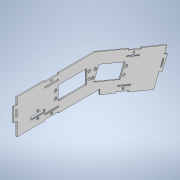
# Autodesk Inventor part: centralFinal
Saved by Autodesk Inventor 2020 (Build 240168000, 168)
## iProperties
Created: 2019-06-16
Part Number: centralFinal
Material: Generic
Document SubType Name: Modeling
Designer: Vivek Muskan
Density: 1 g/cm^3
Appearance: Default
Author: Vivek Muskan
Autodesk Inventor part; units mm, degrees
ref_plane "YZ Plane" through (0, 0, 0) normal (1, 0, 0) x (0, 1, 0)
ref_plane "XZ Plane" through (0, 0, 0) normal (0, 1, 0) x (-1, 0, 0)
ref_plane "XY Plane" through (0, 0, 0) normal (0, 0, 1) x (1, 0, 0)
sketch "Sketch1" plane through (0, 0, 0) normal (1, 0, 0) x (0, 1, 0)
  line L0 (12, -9) -> (2, -9)
  line L1 (2, -9) -> (2, 41)
  line L2 (2, 41) -> (7, 41)
  line L3 (7, 41) -> (7, 31)
  line L4 (7, 31) -> (12, 31)
  line L5 (12, 31) -> (12, -9)
  line L6 (2, 111) -> (12, 111)
  line L7 (12, 111) -> (12, 71)
  line L8 (12, 71) -> (7, 71)
  line L9 (7, 71) -> (7, 61)
  line L10 (7, 61) -> (2, 61)
  line L11 (2, 61) -> (2, 111)
  line L12 (7, 54.5) -> (7, 55)
  line L13 (7, 55) -> (62, 55)
  arc A0 (64, 57) -> (62, 55) centre (64, 55) ccw
  line L14 (64, 57) -> (65, 57)
  arc A1 (67, 55) -> (65, 57) centre (65, 55) ccw
  line L15 (67, 55) -> (102, 55)
  arc A2 (104, 57) -> (102, 55) centre (104, 55) ccw
  line L16 (104, 57) -> (105, 57)
  arc A3 (107, 55) -> (105, 57) centre (105, 55) ccw
  line L17 (107, 55) -> (107, 47)
  arc A4 (105, 45) -> (107, 47) centre (105, 47) ccw
  line L18 (105, 45) -> (104, 45)
  arc A5 (102, 47) -> (104, 45) centre (104, 47) ccw
  line L19 (102, 47) -> (67, 47)
  arc A6 (65, 45) -> (67, 47) centre (65, 47) ccw
  line L20 (65, 45) -> (64, 45)
  arc A7 (62, 47) -> (64, 45) centre (64, 47) ccw
  line L21 (62, 47) -> (7, 47)
  line L22 (7, 47) -> (7, 47.5)
  line L23 (7, 47.5) -> (-5, 47.5)
  line L24 (-5, 47.5) -> (-5, 41)
  line L25 (-5, 41) -> (0, 41)
  line L26 (0, 41) -> (0, 2.0396)
  line L27 (0, 2.0396) -> (0.3922, 1.9612)
  line L28 (0.3922, 1.9612) -> (0, 1.0198)
  line L29 (0, 1.0198) -> (0, 0)
  line L30 (0, 0) -> (-0.3922, 0.0784)
  line L31 (-0.3922, 0.0784) -> (-15.377, -35.885)
  line L32 (-15.377, -35.885) -> (-19.9924, -33.9619)
  line L33 (-19.9924, -33.9619) -> (-22.4924, -39.9619)
  line L34 (-22.4924, -39.9619) -> (-11.4155, -44.5773)
  line L35 (-11.4155, -44.5773) -> (-11.2232, -44.1158)
  line L36 (-11.2232, -44.1158) -> (39.5461, -65.2696)
  arc A8 (42.1615, -64.1927) -> (39.5461, -65.2696) centre (41.3922, -66.0388) ccw
  line L37 (42.1615, -64.1927) -> (43.0845, -64.5773)
  arc A9 (44.1615, -67.1927) -> (43.0845, -64.5773) centre (42.3153, -66.4235) ccw
  line L38 (44.1615, -67.1927) -> (76.4692, -80.6542)
  arc A10 (79.0845, -79.5773) -> (76.4692, -80.6542) centre (78.3153, -81.4235) ccw
  line L39 (79.0845, -79.5773) -> (80.0076, -79.9619)
  arc A11 (81.0845, -82.5773) -> (80.0076, -79.9619) centre (79.2384, -81.8081) ccw
  line L40 (81.0845, -82.5773) -> (78.0076, -89.9619)
  arc A12 (75.3922, -91.0388) -> (78.0076, -89.9619) centre (76.1615, -89.1927) ccw
  line L41 (75.3922, -91.0388) -> (74.4692, -90.6542)
  arc A13 (73.3922, -88.0388) -> (74.4692, -90.6542) centre (75.2384, -88.8081) ccw
  line L42 (73.3922, -88.0388) -> (41.0845, -74.5773)
  arc A14 (38.4692, -75.6542) -> (41.0845, -74.5773) centre (39.2384, -73.8081) ccw
  line L43 (38.4692, -75.6542) -> (37.5461, -75.2696)
  arc A15 (36.4692, -72.6542) -> (37.5461, -75.2696) centre (38.3153, -73.4235) ccw
  line L44 (36.4692, -72.6542) -> (-14.3001, -51.5004)
  line L45 (-14.3001, -51.5004) -> (-14.1078, -51.0388)
  line L46 (-14.1078, -51.0388) -> (-25.1847, -46.4235)
  line L47 (-25.1847, -46.4235) -> (-27.6847, -52.4235)
  line L48 (-27.6847, -52.4235) -> (-23.0693, -54.3465)
  line L49 (-23.0693, -54.3465) -> (-38.8385, -92.1927)
  line L50 (-38.8385, -92.1927) -> (-47.3001, -86.5004)
  line L51 (-47.3001, -86.5004) -> (-30.377, -45.885)
  line L52 (-30.377, -45.885) -> (-39.6078, -42.0388)
  line L53 (-39.6078, -42.0388) -> (-35.7616, -32.8081)
  line L54 (-35.7616, -32.8081) -> (-26.5308, -36.6542)
  line L55 (-26.5308, -36.6542) -> (-10, 3.0198)
  line L56 (-10, 3.0198) -> (-10, 46)
  line L57 (-10, 46) -> (-20, 46)
  line L58 (-20, 46) -> (-20, 56)
  line L59 (-20, 56) -> (-10, 56)
  line L60 (-10, 56) -> (-10, 100)
  line L61 (-10, 100) -> (0, 102)
  line L62 (0, 102) -> (0, 61)
  line L63 (0, 61) -> (-5, 61)
  line L64 (-5, 61) -> (-5, 54.5)
  line L65 (-5, 54.5) -> (7, 54.5)
  line L66 (0, 51) -> (107, 51)
  line L67 (79.5461, -86.2696) -> (-37.6847, -37.4235)
  constraints: 136 end point, 32 point on circle, 16 centre point, 3 midpoint
sketch "Sketch2" plane through (0, 0, 0) normal (1, 0, 0) x (0, 1, 0)
  line L0 (0, 0) -> (0, 51)
  line L1 (0, 51) -> (15, 51)
  line L2 (15, 51) -> (15, 101)
  line L3 (15, 101) -> (65, 101)
  line L4 (101.707, 46.9392) -> (84.707, 46.9392)
  line L5 (84.707, 46.9392) -> (34.707, 46.9392)
  line L6 (15, 51) -> (15, 60)
  line L7 (0, 0) -> (0, 1)
  line L8 (0, 1) -> (110.5886, -21.1178)
  line L9 (50.3822, 41.5) -> (30.3822, 41.5)
  line L10 (30.3822, 41.5) -> (30.3822, 0.5)
  line L11 (30.3822, 0.5) -> (50.3822, 0.5)
  line L12 (50.3822, 0.5) -> (50.3822, 41.5)
  line L13 (50.3822, 0.5) -> (45.3822, 0.5)
  line L14 (45.3822, 0.5) -> (45.3822, -3.5)
  line L15 (45.3822, -3.5) -> (35.3822, -3.5)
  circle A0 centre (45.3822, -3.5) radius 2
  circle A1 centre (35.3822, -3.5) radius 2
  line L16 (50.3822, 21) -> (30.3822, 21)
  circle A2 centre (45.3822, 45.5) radius 2
  circle A3 centre (35.3822, 45.5) radius 2
  line L17 (65, 101) -> (65, -12.0001)
  line L18 (0, 51) -> (107.1279, 51)
  line L19 (65, 51) -> (55, 51)
  line L20 (15, 51) -> (25, 51)
  line L21 (-5.3847, -50.9231) -> (-24.6156, -97.0769)
  line L22 (-24.6156, -97.0769) -> (21.5382, -116.3077)
  line L23 (21.5382, -116.3077) -> (65, -12.0001)
  line L24 (15, 51) -> (15, -19)
  line L25 (-5.3847, -50.9231) -> (7.9166, -19)
  line L26 (15, -19) -> (7.9166, -19)
  line L27 (30.9296, -55.7624) -> (12.468, -48.0701)
  line L28 (12.468, -48.0701) -> (28.2374, -10.224)
  line L29 (28.2374, -10.224) -> (46.6989, -17.9163)
  line L30 (46.6989, -17.9163) -> (30.9296, -55.7624)
  circle A4 centre (43.622, -12.3009) radius 2
  circle A5 centre (34.3912, -8.4548) radius 2
  circle A6 centre (24.7757, -57.5317) radius 2
  circle A7 centre (15.545, -53.6855) radius 2
  line L31 (65, 51) -> (65, 41)
  line L32 (65, 41) -> (63.5, 41)
  line L33 (63.5, 41) -> (63.5, 61)
  line L34 (63.5, 61) -> (65, 61)
  line L35 (65, 61) -> (65, 41)
  line L36 (63.5, 61) -> (57.5, 61)
  line L37 (57.5, 61) -> (56, 61)
  line L38 (56, 61) -> (56, 41)
  line L39 (56, 41) -> (57.5, 41)
  line L40 (57.5, 41) -> (57.5, 61)
  line L41 (65, 51) -> (60.5, 51)
  circle A8 centre (60.5, 51) radius 1.5
  line L42 (44.6152, -60.9232) -> (43.2306, -60.3463)
  line L43 (43.2306, -60.3463) -> (35.5383, -78.8078)
  line L44 (35.5383, -78.8078) -> (36.9229, -79.3847)
  line L45 (29.9998, -76.5001) -> (28.6152, -75.9231)
  line L46 (28.6152, -75.9231) -> (36.3076, -57.4616)
  line L47 (36.3076, -57.4616) -> (37.6922, -58.0386)
  line L48 (37.6922, -58.0386) -> (29.9998, -76.5001)
  circle A9 centre (36.6152, -68.4232) radius 1.5
  line L49 (-1.5387, -106.6923) -> (40, -7)
  line L50 (40, 101) -> (40, -7)
  line L51 (40, -68.0997) -> (40, -71.9997)
  circle A10 centre (-1.2309, -52.6538) radius 1.5
  line L52 (5.3845, -44.5769) -> (-2.3078, -63.0385)
  line L53 (-0.9232, -63.6154) -> (6.7691, -45.1539)
  line L54 (6.7691, -45.1539) -> (5.3845, -44.5769)
  line L55 (-2.3078, -63.0385) -> (-0.9232, -63.6154)
  line L56 (-0.1539, -42.2692) -> (-7.8463, -60.7308)
  line L57 (-7.8463, -60.7308) -> (-9.2309, -60.1538)
  line L58 (-1.5386, -41.6923) -> (-0.1539, -42.2692)
  line L59 (15, 41) -> (16.5, 41)
  line L60 (16.5, 41) -> (16.5, 61)
  line L61 (16.5, 61) -> (15, 61)
  line L62 (22.5, 61) -> (24, 61)
  line L63 (24, 61) -> (24, 41)
  line L64 (24, 41) -> (22.5, 41)
  line L65 (22.5, 41) -> (22.5, 61)
  circle A11 centre (19.5, 51) radius 1.5
  dimension "d0" = 51
  dimension "d1" = 15
  dimension "d2" = 50
  dimension "d3" = 50
  dimension "d11" = 17
  dimension "d12" = 50
  dimension "d23" = 9
  dimension "d34" = 1
  dimension "d35" = 78.69
  dimension "d36" = 20
  dimension "d37" = 41
  dimension "d38" = 5
  dimension "d39" = 4
  dimension "d40" = 10
  dimension "d41" = 4
  dimension "d42" = 4
  dimension "d43" = 10
  dimension "d47" = 10
  dimension "d48" = 70
  dimension "d86" = 10
  dimension "d87" = 1.5
  dimension "d88" = 20
  dimension "d89" = 6
  dimension "d90" = 1.5
  dimension "d91" = 20
  dimension "d92" = 4.5
  dimension "d93" = 3
  constraints: 132 end point, 40 symmetric about line, 14 point on line, 12 centre point, 8 horizontal, 7 perpendicular, 6 parallel, 5 vertical, 4 midpoint, 3 coincident, 9 other
  measures "d0" distance of L0.start L0.end
  measures "d1" distance of L0.end L1.end
  measures "d2" distance of L1.end L2.end
  measures "d3" distance of L2.end L3.end
  measures "d11" distance of L4.start L4.end
  measures "d12" distance of L4.end L5.end
  measures "d23" distance of L1.end L6.end
  measures "d34" distance of L0.start L7.end
  measures "d35" angle of L7 L8
  measures "d36" distance of L11.end L10.end
  measures "d37" distance of L10.end L9.end
  measures "d38" distance of L11.end L13.end
  measures "d39" distance of L13.end L14.end
  measures "d40" distance of L14.end L15.end
  measures "d41" diameter of A0
  measures "d42" diameter of A1
  measures "d43" distance of L19.start L19.end
  measures "d47" distance of L1.end L20.end
  measures "d48" distance of L1.end L24.end
  measures "d86" distance of L19.start L31.end
  measures "d87" distance of L33.end L34.end
  measures "d88" distance of L32.end L33.end
  measures "d89" distance of L33.end L36.end
  measures "d90" distance of L39.end L38.end
  measures "d91" distance of L38.end L37.end
  measures "d92" distance of L19.start L41.end
  measures "d93" diameter of A8
extrude "Extrusion1" add sketch "Sketch2" along normal blind 1.5 contours L24 L59 L60 L18 A11 L65 L64 L63 L50 L9 L10 L11 L8 | L8 L49 L29 L28 L27 L22 L21 L57 L56 L58 L25 L26 L24 | L2 L61 L60 L18 | L18 L60 L59 L24 | L50 L15 A0 L14 L11 L12 L9 L5 A2 L38 L39 L40 L33 L32 L17 L8 | L8 L23 L42 L43 L44 L22 L49 L27 L30 L29 | L60 L61 L2 L3 L50 L18 L63 L62 L65 A11 | L50 L11 L14 A0 L15 | A11 L18 | L18 A11 | L32 L33 L5 L17 | L23 L51 L43 L42 | L58 L56 L57 L21 L25 | L5 L33 L18 L17 | L23 L44 L43 L51 | L3 L17 L34 L36 L37 L38 L18 L50 | L65 L62 L63 L18 | L18 L63 L64 L65 | L5 L40 L18 A8 L33 | L18 L33 L34 L17 | L18 L38 L5 A2 L50 | L40 L39 L38 L5 | L5 L38 L18 L40 | L18 A8 L40 L36 L33 | L18 L38 L37 L40 | A8 L18 | L18 A8 | L45 L46 L47 L48 | A9 | A10 | L54 L53 L55 L52
sketch "Sketch3" plane through (1.5, 0, 0) normal (1, 0, 0) x (0, 0, -1)
  line L0 (-101, 65) -> (-101, 15) projected
  line L1 (-101, 65) -> (-101, 55)
  line L2 (-101, 55) -> (-106, 55)
  line L3 (-106, 55) -> (-106, 35)
  line L4 (-106, 35) -> (-101, 35)
  line L5 (-101, 55) -> (-101, 50)
  line L6 (-101, 50) -> (-102.5, 50)
  line L7 (-102.5, 50) -> (-102.5, 40)
  line L8 (-102.5, 40) -> (-101, 40)
  line L9 (-101, 40) -> (-101, 50)
  line L10 (-1, 0) -> (21.1178, 110.5886) projected
  line L11 (116.3077, 21.5382) -> (97.0769, -24.6156)
  line L12 (112.4616, 12.3074) -> (117.0769, 10.3843)
  line L13 (117.0769, 10.3843) -> (109.3846, -8.0772)
  line L14 (109.3846, -8.0772) -> (104.7692, -6.1541)
  line L15 (110.5385, 7.692) -> (111.9231, 7.1151)
  line L16 (111.9231, 7.1151) -> (108.0769, -2.1156)
  line L17 (108.0769, -2.1156) -> (106.6923, -1.5387)
  point P0 (0, 0)
  point P1 (106.6923, -1.5387)
  dimension "d66" = 10
  dimension "d67" = 5
  dimension "d68" = 20
  dimension "d69" = 5
  dimension "d70" = 1.5
  dimension "d71" = 10
  constraints: 32 end point, 10 symmetric about line, 6 point on line, 4 perpendicular, 2 parallel, 1 horizontal
  measures "d66" distance of L0.start L1.end
  measures "d67" distance of L1.end L2.end
  measures "d68" distance of L2.end L3.end
  measures "d69" distance of L1.end L5.end
  measures "d70" distance of L8.end L7.end
  measures "d71" distance of L7.end L6.end
extrude "Extrusion2" add sketch "Sketch3" against normal blind 1.5 contours L0 L6 L7 L8 L4 L3 L2
extrude "Extrusion3" add sketch "Sketch3" against normal blind 1.5 contours L12 L13 L14 L11 L17 L16 L15
sketch "Sketch4" plane through (1.5, 0, 0) normal (1, 0, 0) x (0, 0, -1)
  line L0 (-101, 15) -> (19, 15) projected
  line L1 (-101, 15) -> (-101, 30)
  line L2 (-101, 35) -> (-101, 15) projected
  line L3 (-101, 30) -> (-81, 30)
  line L4 (-81, 30) -> (-61, 30)
  line L5 (-61, 30) -> (-61, 26)
  line L6 (-61, 26) -> (-81, 26)
  line L7 (-81, 26) -> (-81, 30)
  line L8 (-71, 30) -> (-71, 33)
  line L9 (-71, 33) -> (-71, 23)
  circle A0 centre (-71, 33) radius 1.5
  circle A1 centre (-71, 23) radius 1.5
  point P0 (0, 0)
  dimension "d76" = 15
  dimension "d77" = 20
  dimension "d78" = 20
  dimension "d79" = 4
  dimension "d80" = 3
  dimension "d81" = 10
  dimension "d82" = 3
  dimension "d83" = 3
  constraints: 16 end point, 2 centre point, 2 coincident, 2 horizontal, 2 parallel, 2 point on line, 1 midpoint, 1 perpendicular, 1 vertical
  measures "d76" distance of L0.start L1.end
  measures "d77" distance of L1.end L3.end
  measures "d78" distance of L5.end L6.end
  measures "d79" distance of L4.end L5.end
  measures "d80" distance of L8.start L8.end
  measures "d81" distance of L8.end L9.end
  measures "d82" diameter of A0
  measures "d83" diameter of A1
extrude "Extrusion6" cut sketch "Sketch2" along normal blind 1.5 contours L2 L61 L60 L18 | L18 L60 L59 L24 | A11 L18 | L18 A11 | L32 L33 L5 L17 | L58 L56 L57 L21 L25 | L5 L33 L18 L17 | L65 L62 L63 L18 | L18 L63 L64 L65 | L18 L33 L34 L17 | L40 L39 L38 L5 | L5 L38 L18 L40 | L18 L38 L37 L40 | A8 L18 | L18 A8 | A10 | L54 L53 L55 L52
extrude "Extrusion7" cut sketch "Sketch2" along normal blind 1.5 contours L23 L51 L43 L42 | L23 L44 L43 L51 | L45 L46 L47 L48 | A9
extrude "Extrusion8" cut sketch "Sketch4" against normal blind 1.5 contours A0 | L4 L9 L6 L7 | L4 L5 L6 L9
extrude "Extrusion9" cut sketch "Sketch4" against normal blind 10 contours A1
body "Solid1"
